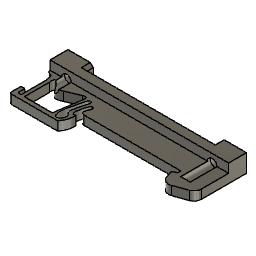
DIN_Rail_RPi3B+_v17 (Autodesk Fusion 360 design; units mm, degrees)
Autodesk Fusion 360 part; units mm, degrees
sketch "Skizze1" plane through (0, 0, 0) normal (0, 0, 1) x (1, 0, 0)
  line L0 (-18.504, -16.9705) -> (15.5063, -16.9705)
  line L1 (15.5063, -16.9705) -> (15.5063, -18.0189)
  line L2 (15.5063, -18.0189) -> (14.1084, -18.7179)
  line L3 (14.1084, -18.7179) -> (15.6525, -23.606)
  line L4 (15.6525, -23.606) -> (24.227, -20.5719)
  line L5 (-35.9646, -23.0715) -> (-19.7137, -23.0715)
  line L6 (-18.504, -16.9705) -> (-17.2228, -13.4469)
  line L7 (-17.2228, -13.4469) -> (-17.946, -13.1839)
  line L8 (-19.2954, -18.4641) -> (-18.2688, -18.4641)
  line L9 (-35.9646, -23.0715) -> (-35.9646, -19.2117)
  line L10 (-35.9646, -19.2117) -> (-34.6452, -19.2117)
  line L11 (-34.6452, -19.2117) -> (-34.6452, -21.6588)
  line L12 (-34.6452, -21.6588) -> (-33.5347, -21.6588)
  line L13 (-33.5347, -21.6588) -> (-33.5347, -13.2264)
  line L14 (-33.5347, -13.2264) -> (-34.0899, -10.632)
  line L15 (-32.3923, -21.6588) -> (-23.0123, -21.6588)
  line L16 (-23.0123, -21.6588) -> (-21.6594, -12.669)
  line L17 (-22.9169, -11.5274) -> (-27.4008, -13.4467)
  line L18 (-32.3923, -13.2264) -> (-32.3923, -21.6588)
  spline S0 degree 5 poles (-19.2954, -18.4641) (-19.3184, -18.3927) (-19.3603, -18.2542) (-19.4104, -18.0594) (-19.4525, -17.8207) (-19.4675, -17.5308) (-19.4493, -17.2185) (-19.4029, -16.8572) (-19.3324, -16.4356) (-19.241, -15.9625) (-19.1312, -15.4589) (-19.0048, -14.9531) (-18.8629, -14.4755) (-18.7064, -14.0535) (-18.5361, -13.7054) (-18.3528, -13.4397) (-18.1961, -13.2951) (-18.0732, -13.2248) (-17.9888, -13.1947) (-17.946, -13.1839) knots 0 0 0 0 0 0 0.066667 0.133333 0.2 0.266667 0.333333 0.4 0.466667 0.533333 0.6 0.666667 0.733333 0.8 0.866667 0.933333 1 1 1 1 1 1
  spline S1 degree 5 poles (-18.2688, -18.4641) (-18.2632, -18.5566) (-18.2552, -18.7417) (-18.2522, -19.0191) (-18.2669, -19.3888) (-18.3183, -19.8506) (-18.4055, -20.312) (-18.5313, -20.7729) (-18.6968, -21.2334) (-18.9, -21.6935) (-19.1378, -22.1532) (-19.3534, -22.5207) (-19.5285, -22.7962) (-19.651, -22.9798) (-19.7137, -23.0715) knots 0 0 0 0 0 0 0.1 0.2 0.3 0.4 0.5 0.6 0.7 0.8 0.9 1 1 1 1 1 1
  spline S2 degree 5 poles (-32.3923, -13.2264) (-32.4041, -13.159) (-32.4253, -13.0268) (-32.4498, -12.8368) (-32.4679, -12.6002) (-32.4661, -12.3331) (-32.4399, -12.0964) (-32.3897, -11.8934) (-32.3162, -11.7295) (-32.221, -11.612) (-32.106, -11.5486) (-31.9731, -11.5456) (-31.8242, -11.6057) (-31.661, -11.7275) (-31.4857, -11.906) (-31.3014, -12.1335) (-31.1123, -12.3991) (-30.924, -12.6899) (-30.7407, -12.991) (-30.5632, -13.2862) (-30.3877, -13.5586) (-30.2028, -13.7909) (-29.9878, -13.9661) (-29.7146, -14.0679) (-29.3521, -14.0813) (-28.8695, -13.9935) (-28.3658, -13.8341) (-27.9133, -13.6614) (-27.5773, -13.5222) (-27.4008, -13.4467) knots 0 0 0 0 0 0 0.04 0.08 0.12 0.16 0.2 0.24 0.28 0.32 0.36 0.4 0.44 0.48 0.52 0.56 0.6 0.64 0.68 0.72 0.76 0.8 0.84 0.88 0.92 0.96 1 1 1 1 1 1
  line L19 (-19.0879, -19.1073) -> (-19.5029, -17.8209)
  spline S3 degree 5 poles (-19.3635, -12.5816) (-19.3584, -12.5314) (-19.3535, -12.4353) (-19.3628, -12.3041) (-19.4111, -12.152) (-19.5309, -11.9952) (-19.7024, -11.8756) (-19.9083, -11.8159) (-20.1258, -11.8493) (-20.3333, -12.0055) (-20.5179, -12.289) (-20.6789, -12.6934) (-20.8232, -13.2083) (-20.9619, -13.8182) (-21.1069, -14.5045) (-21.2679, -15.2461) (-21.4472, -16.0207) (-21.6395, -16.8063) (-21.8218, -17.5812) (-21.9666, -18.3279) (-22.063, -19.0362) (-22.1058, -19.6988) (-22.0967, -20.3096) (-22.0398, -20.8619) (-21.9398, -21.3449) (-21.8, -21.7438) (-21.6173, -22.0324) (-21.3849, -22.1819) (-21.124, -22.2225) (-20.8611, -22.1978) (-20.621, -22.1483) (-20.4106, -22.0779) (-20.2225, -21.9626) (-20.046, -21.7734) (-19.8749, -21.4944) (-19.717, -21.1435) (-19.5887, -20.7596) (-19.509, -20.3887) (-19.4941, -20.0709) (-19.5517, -19.8273) (-19.6746, -19.6452) (-19.8452, -19.4912) (-20.0397, -19.3271) (-20.2337, -19.1261) (-20.406, -18.8851) (-20.54, -18.6143) (-20.625, -18.33) (-20.6578, -18.0459) (-20.644, -17.7643) (-20.5955, -17.4786) (-20.5263, -17.1782) (-20.4491, -16.852) (-20.371, -16.4934) (-20.2925, -16.1023) (-20.2097, -15.6834) (-20.1175, -15.245) (-20.0112, -14.798) (-19.8891, -14.3547) (-19.7554, -13.9273) (-19.6204, -13.5272) (-19.4978, -13.1637) (-19.4219, -12.9078) (-19.3839, -12.7367) (-19.3685, -12.6318) (-19.3635, -12.5816) knots 0 0 0 0 0 0 0.01666667 0.03333333 0.05 0.06666667 0.08333333 0.1 0.11666667 0.13333333 0.15 0.16666667 0.18333333 0.2 0.21666667 0.23333333 0.25 0.26666667 0.28333333 0.3 0.31666667 0.33333333 0.35 0.36666667 0.38333333 0.4 0.41666667 0.43333333 0.45 0.46666667 0.48333333 0.5 0.51666667 0.53333333 0.55 0.56666667 0.58333333 0.6 0.61666667 0.63333333 0.65 0.66666667 0.68333333 0.7 0.71666667 0.73333333 0.75 0.76666667 0.78333333 0.8 0.81666667 0.83333333 0.85 0.86666667 0.88333333 0.9 0.91666667 0.93333333 0.95 0.96666667 0.98333333 1 1 1 1 1 1
  line L20 (-19.8268, -11.5696) -> (-20.7201, -12.3941)
  spline S4 degree 5 poles (-21.6594, -12.669) (-21.643, -12.5969) (-21.6137, -12.4571) (-21.5807, -12.2601) (-21.5587, -12.0237) (-21.5707, -11.7747) (-21.6255, -11.5766) (-21.7267, -11.4334) (-21.8764, -11.3476) (-22.0728, -11.317) (-22.3123, -11.3376) (-22.5356, -11.3916) (-22.7199, -11.4519) (-22.85, -11.5008) (-22.9169, -11.5274) knots 0 0 0 0 0 0 0.1 0.2 0.3 0.4 0.5 0.6 0.7 0.8 0.9 1 1 1 1 1 1
  line L21 (-28.7659, -14.031) -> (-26.0357, -12.8623)
  line L22 (-21.291, -15.345) -> (-22.0046, -18.3535)
  line L23 (-22.1274, -21.141) -> (-21.3425, -22.4993)
  line L24 (-34.0899, -10.632) -> (-35.773, -10.632)
  line L25 (-35.773, -10.632) -> (-35.773, -3.632)
  line L26 (-35.773, -3.632) -> (24.227, -3.632)
  line L27 (24.227, -3.632) -> (24.227, -20.5719)
  point P0 (-19.4161, -16.9785)
  point P1 (-18.7883, -14.2872)
  point P2 (-18.5219, -20.7105)
  point P3 (-32.3923, -11.9292)
  point P4 (-32.0431, -11.555)
  point P5 (-31.3695, -12.0539)
  point P6 (-30.3467, -13.6006)
  point P7 (-19.5978, -11.9589)
  point P8 (-20.2735, -11.9818)
  point P9 (-21.6478, -16.8493)
  point P10 (-21.7349, -21.8202)
  point P11 (-20.7944, -22.1798)
  point P12 (-20.0435, -21.7459)
  point P13 (-19.5147, -20.06)
  point P14 (-20.0074, -19.3484)
  point P15 (-20.6205, -18.2864)
  point P16 (-20.4782, -16.9727)
  point P17 (-19.9417, -14.5531)
  point P18 (-21.7422, -11.4446)
  dimension "d1" = 60
  dimension "d2" = 7
  constraint horizontal L0
  constraint perpendicular L0 L1
  constraint horizontal L5
  constraint perpendicular L6 L7
  constraint perpendicular L5 L9
  constraint perpendicular L9 L10
  constraint perpendicular L10 L11
  constraint perpendicular L9 L12
  constraint perpendicular L10 L13
  constraint perpendicular L9 L15
  constraint perpendicular L15 L18
  constraint midpoint L8.start L19
  constraint midpoint P8 L20
  constraint midpoint L17.end L21
  constraint coincident L17 L21.end
  constraint midpoint P9 L22
  constraint midpoint P10 L23
  constraint perpendicular L13 L24
  constraint perpendicular L24 L25
  constraint perpendicular L25 L26
  constraint perpendicular L26 L27
  measures "d1" distance of L25.end L26.end
  measures "d2" distance of L24.end L25.end
extrude "Extrusion1" add sketch "Skizze1" along normal blind 3
fillet "Abrundung1" radius 1 1 edges at (-18.504, -16.9705, 1.5)
fillet "Abrundung2" radius 0.5 1 edges at (-17.2228, -13.4469, 1.5)
fillet "Abrundung3" radius 0.5 3 edges at (-35.9646, -23.0715, 1.5) (-34.6452, -21.6588, 1.5) (-33.5347, -21.6588, 1.5)
fillet "Abrundung4" radius 1 3 edges at (-33.5347, -13.2264, 1.5) (-34.0899, -10.632, 1.5) (-35.773, -10.632, 1.5)
fillet "Abrundung5" radius 2.5 2 edges at (15.6525, -23.606, 1.5) (24.227, -20.5719, 1.5)
sketch "Skizze2" plane through (0, 0, 3) normal (0, 0, 1) x (-1, 0, 0)
  arc A0 (-22.5609, 21.1614) -> (-24.227, 18.8046) centre (-21.727, 18.8046) ccw
  line L0 (-24.227, 18.8046) -> (-24.227, 3.632)
  line L1 (-24.227, 3.632) -> (35.773, 3.632)
  line L2 (35.773, 3.632) -> (35.773, 9.6359)
  arc A1 (35.773, 9.6359) -> (34.8358, 10.6339) centre (34.773, 9.6359) ccw
  arc A2 (33.9207, 11.4227) -> (34.8358, 10.6339) centre (34.8986, 11.632) ccw
  line L3 (33.9207, 11.4227) -> (33.5569, 13.123)
  arc A3 (33.5347, 13.3322) -> (33.5569, 13.123) centre (34.5347, 13.3322) ccw
  line L4 (33.5347, 13.3322) -> (33.5347, 21.1588)
  arc A4 (34.0347, 21.6588) -> (33.5347, 21.1588) centre (34.0347, 21.1588) ccw
  line L5 (34.0347, 21.6588) -> (34.1452, 21.6588)
  arc A5 (34.6452, 21.1588) -> (34.1452, 21.6588) centre (34.1452, 21.1588) ccw
  line L6 (34.6452, 21.1588) -> (34.6452, 19.2117)
  line L7 (34.6452, 19.2117) -> (35.9646, 19.2117)
  line L8 (35.9646, 19.2117) -> (35.9646, 22.5715)
  arc A6 (35.9646, 22.5715) -> (35.4646, 23.0715) centre (35.4646, 22.5715) ccw
  line L9 (35.4646, 23.0715) -> (19.7137, 23.0715)
  spline S0 degree 5 poles (19.7137, 23.0715) (19.651, 22.9798) (19.5285, 22.7962) (19.3534, 22.5207) (19.1378, 22.1532) (18.9, 21.6935) (18.6968, 21.2334) (18.5313, 20.7729) (18.4055, 20.312) (18.3183, 19.8506) (18.2669, 19.3888) (18.2522, 19.0191) (18.2552, 18.7417) (18.2632, 18.5566) (18.2688, 18.4641) knots -1 -1 -1 -1 -1 -1 -0.9 -0.8 -0.7 -0.6 -0.5 -0.4 -0.3 -0.2 -0.1 0 0 0 0 0 0
  line L10 (18.2688, 18.4641) -> (19.2954, 18.4641)
  spline S1 degree 5 poles (19.2954, 18.4641) (19.3184, 18.3927) (19.3603, 18.2542) (19.4104, 18.0594) (19.4525, 17.8207) (19.4675, 17.5308) (19.4493, 17.2185) (19.4029, 16.8572) (19.3324, 16.4356) (19.241, 15.9625) (19.1312, 15.4589) (19.0048, 14.9531) (18.8629, 14.4755) (18.7064, 14.0535) (18.5361, 13.7054) (18.3528, 13.4397) (18.1961, 13.2951) (18.0732, 13.2248) (17.9888, 13.1947) (17.946, 13.1839) knots 0 0 0 0 0 0 0.066667 0.133333 0.2 0.266667 0.333333 0.4 0.466667 0.533333 0.6 0.666667 0.733333 0.8 0.866667 0.933333 1 1 1 1 1 1
  line L11 (17.946, 13.1839) -> (17.6927, 13.276)
  arc A7 (17.3936, 13.9168) -> (17.6927, 13.276) centre (17.8635, 13.7459) ccw
  line L12 (17.3936, 13.9168) -> (18.0161, 15.6288)
  arc A8 (18.0161, 15.6288) -> (17.0763, 16.9705) centre (17.0763, 15.9705) ccw
  line L13 (17.0763, 16.9705) -> (-15.5063, 16.9705)
  line L14 (-15.5063, 16.9705) -> (-15.5063, 18.0189)
  line L15 (-15.5063, 18.0189) -> (-14.1084, 18.7179)
  line L16 (-14.1084, 18.7179) -> (-14.8733, 21.1393)
  arc A9 (-14.8733, 21.1393) -> (-18.0911, 22.7431) centre (-17.2572, 20.3863) ccw
  line L17 (-18.0911, 22.7431) -> (-22.5609, 21.1614)
  line L18 (32.3923, 21.6588) -> (32.3923, 13.2264)
  spline S2 degree 5 poles (32.3923, 13.2264) (32.4041, 13.159) (32.4253, 13.0268) (32.4498, 12.8368) (32.4679, 12.6002) (32.4661, 12.3331) (32.4399, 12.0964) (32.3897, 11.8934) (32.3162, 11.7295) (32.221, 11.612) (32.106, 11.5486) (31.9731, 11.5456) (31.8242, 11.6057) (31.661, 11.7275) (31.4857, 11.906) (31.3014, 12.1335) (31.1123, 12.3991) (30.924, 12.6899) (30.7407, 12.991) (30.5632, 13.2862) (30.3877, 13.5586) (30.2028, 13.7909) (29.9878, 13.9661) (29.7146, 14.0679) (29.3521, 14.0813) (28.8695, 13.9935) (28.3658, 13.8341) (27.9133, 13.6614) (27.5773, 13.5222) (27.4008, 13.4467) knots 0 0 0 0 0 0 0.04 0.08 0.12 0.16 0.2 0.24 0.28 0.32 0.36 0.4 0.44 0.48 0.52 0.56 0.6 0.64 0.68 0.72 0.76 0.8 0.84 0.88 0.92 0.96 1 1 1 1 1 1
  line L19 (27.4008, 13.4467) -> (22.9169, 11.5274)
  spline S3 degree 5 poles (22.9169, 11.5274) (22.85, 11.5008) (22.7199, 11.4519) (22.5356, 11.3916) (22.3123, 11.3376) (22.0728, 11.317) (21.8764, 11.3476) (21.7267, 11.4334) (21.6255, 11.5766) (21.5707, 11.7747) (21.5587, 12.0237) (21.5807, 12.2601) (21.6137, 12.4571) (21.643, 12.5969) (21.6594, 12.669) knots -1 -1 -1 -1 -1 -1 -0.9 -0.8 -0.7 -0.6 -0.5 -0.4 -0.3 -0.2 -0.1 0 0 0 0 0 0
  line L20 (21.6594, 12.669) -> (23.0123, 21.6588)
  line L21 (23.0123, 21.6588) -> (32.3923, 21.6588)
  spline S4 degree 5 poles (19.3635, 12.5816) (19.3685, 12.6318) (19.3839, 12.7367) (19.4219, 12.9078) (19.4978, 13.1637) (19.6204, 13.5272) (19.7554, 13.9273) (19.8891, 14.3547) (20.0112, 14.798) (20.1175, 15.245) (20.2097, 15.6834) (20.2925, 16.1023) (20.371, 16.4934) (20.4491, 16.852) (20.5263, 17.1782) (20.5955, 17.4786) (20.644, 17.7643) (20.6578, 18.0459) (20.625, 18.33) (20.54, 18.6143) (20.406, 18.8851) (20.2337, 19.1261) (20.0397, 19.3271) (19.8452, 19.4912) (19.6746, 19.6452) (19.5517, 19.8273) (19.4941, 20.0709) (19.509, 20.3887) (19.5887, 20.7596) (19.717, 21.1435) (19.8749, 21.4944) (20.046, 21.7734) (20.2225, 21.9626) (20.4106, 22.0779) (20.621, 22.1483) (20.8611, 22.1978) (21.124, 22.2225) (21.3849, 22.1819) (21.6173, 22.0324) (21.8, 21.7438) (21.9398, 21.3449) (22.0398, 20.8619) (22.0967, 20.3096) (22.1058, 19.6988) (22.063, 19.0362) (21.9666, 18.3279) (21.8218, 17.5812) (21.6395, 16.8063) (21.4472, 16.0207) (21.2679, 15.2461) (21.1069, 14.5045) (20.9619, 13.8182) (20.8232, 13.2083) (20.6789, 12.6934) (20.5179, 12.289) (20.3333, 12.0055) (20.1258, 11.8493) (19.9083, 11.8159) (19.7024, 11.8756) (19.5309, 11.9952) (19.4111, 12.152) (19.3628, 12.3041) (19.3535, 12.4353) (19.3584, 12.5314) (19.3635, 12.5816) knots -1 -1 -1 -1 -1 -1 -0.98333333 -0.96666667 -0.95 -0.93333333 -0.91666667 -0.9 -0.88333333 -0.86666667 -0.85 -0.83333333 -0.81666667 -0.8 -0.78333333 -0.76666667 -0.75 -0.73333333 -0.71666667 -0.7 -0.68333333 -0.66666667 -0.65 -0.63333333 -0.61666667 -0.6 -0.58333333 -0.56666667 -0.55 -0.53333333 -0.51666667 -0.5 -0.48333333 -0.46666667 -0.45 -0.43333333 -0.41666667 -0.4 -0.38333333 -0.36666667 -0.35 -0.33333333 -0.31666667 -0.3 -0.28333333 -0.26666667 -0.25 -0.23333333 -0.21666667 -0.2 -0.18333333 -0.16666667 -0.15 -0.13333333 -0.11666667 -0.1 -0.08333333 -0.06666667 -0.05 -0.03333333 -0.01666667 0 0 0 0 0 0
  line L22 (35.773, 3.632) -> (35.773, 9.632)
  line L23 (-24.227, 3.632) -> (-24.227, 9.632)
  line L24 (-24.227, 9.632) -> (35.773, 9.6359)
  dimension "d11" = 6
  dimension "d12" = 6
  constraint coincident L1.end L2.start
  constraint perpendicular L1 L22
  constraint coincident L0.end L1.start
  constraint perpendicular L1 L23
  constraint coincident L2.end A1.start
  measures "d11" distance of L1.end L22.end
  measures "d12" distance of L0.end L23.end
extrude "Extrusion3" add sketch "Skizze2" along normal blind 3 contours L0 L1 L2 L22 L23 L24
sketch "Skizze3" plane through (0, -3.632, 0) normal (0, 1, 0) x (-1, 0, 0)
  line L0 (-24.227, 0) -> (35.773, 0)
  line L1 (35.773, 0) -> (35.773, 6)
  line L2 (35.773, 6) -> (-24.227, 6)
  line L3 (-24.227, 6) -> (-24.227, 0)
  circle A0 centre (-18.727, 3) radius 1.6
  circle A1 centre (30.273, 3) radius 1.6
  circle A2 centre (-18.727, 3) radius 2
  circle A3 centre (30.273, 3) radius 2
  line L4 (-15.727, 6) -> (-15.727, 0)
  line L5 (27.273, 6) -> (27.273, 0)
  point P0 (-24.227, 3)
  dimension "d27" = 3.2
  dimension "d28" = 3.2
  dimension "d29" = 49
  dimension "d30" = 5.5
  dimension "d31" = 4
  dimension "d32" = 4
  dimension "d37" = 3
  dimension "d38" = 3
  constraint midpoint L3 P0
  constraint horizontal A0.centre P0
  constraint horizontal A1.centre P0
  constraint concentric A0 A2
  constraint concentric A1 A3
  constraint coincident L2 L4.start
  constraint coincident L0 L4.end
  constraint coincident L2 L5.start
  constraint coincident L0 L5.end
  constraint vertical L5
  constraint vertical L4
  measures "d27" diameter of A0
  measures "d28" diameter of A1
  measures "d29" distance of A0.centre A1.centre
  measures "d30" distance of A0.centre P0
  measures "d31" diameter of A2
  measures "d32" diameter of A3
  measures "d37" distance of A0.centre L4
  measures "d38" distance of A1.centre L5
extrude "Extrusion4" cut sketch "Skizze3" against normal blind 5 contours A0 | A1 | A2 | A3
extrude "Extrusion5" cut sketch "Skizze3" against normal blind 15 contours A0 | A1
extrude "Extrusion6" cut sketch "Skizze3" against normal blind 3 contours L0 L2 L4 L5
chamfer "Fase1" distance 1 angle 45 4 edges at (15.727, -5.132, 0) (15.727, -5.132, 6) (-27.273, -5.132, 6) (-27.273, -5.132, 0)
equation "d30 = ( 11 / 2 ) * 1 mm"
named bodies: "DIN_Rail_RPi3B+"
